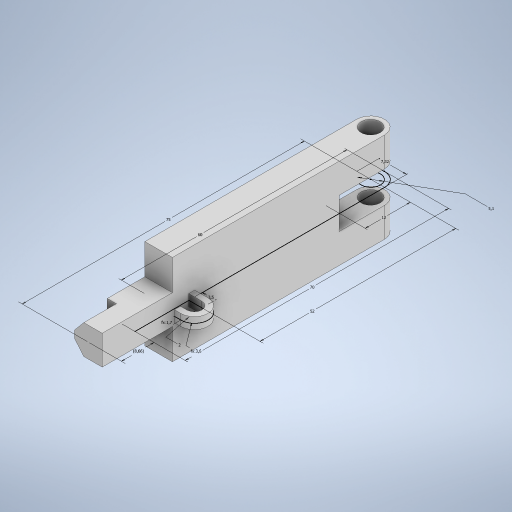
# Autodesk Inventor part: kredafullv3
Saved by Autodesk Inventor 2023 (Build 270158000, 158)
## iProperties
Created: 2023-03-10
Part Number: kredafullv3
Material: Ogólny
Document SubType Name: Modeling
Designer: kamil
Density: 1 g/cm^3
Appearance: Domyślna
Author: kamil
Autodesk Inventor part; units mm, degrees
ref_plane "YZ Plane" through (0, 0, 0) normal (1, 0, 0) x (0, 1, 0)
ref_plane "XZ Plane" through (0, 0, 0) normal (0, 1, 0) x (-1, 0, 0)
ref_plane "XY Plane" through (0, 0, 0) normal (0, 0, 1) x (1, 0, 0)
sketch "Szkic1" plane through (0, 0, 0) normal (0, 1, 0) x (-1, 0, 0)
  line L0 (-3.66, 66.34) -> (-3.66, 0)
  line L1 (-3.66, 0) -> (3.66, 0) construction
  line L2 (3.66, 0) -> (3.66, 66.34)
  arc A0 (-3.66, 0) -> (3.66, 0) centre (0, 0) ccw
  circle A1 centre (0, 0) radius 2.55
  line L3 (3.66, 12) -> (-3.66, 12)
  line L4 (3.66, 66.34) -> (-3.66, 66.34)
  line L5 (3.66, 56.34) -> (-3.66, 56.34)
  line L6 (0, 66.34) -> (0, 75) construction
  line L7 (-3.66, 52) -> (-7.16, 52)
  line L8 (-7.16, 52) -> (-7.16, 50.4)
  line L9 (-7.16, 50.4) -> (-3.66, 50.4)
  line L10 (-3.66, 50.4) -> (-3.66, 52)
  arc A2 (-7.16, 57.6) -> (-7.16, 50.4) centre (-7.16, 54) ccw
  arc A3 (-7.16, 56) -> (-7.16, 52) centre (-7.16, 54) ccw
  line L11 (-7.16, 57.6) -> (-5.46, 57.6)
  line L12 (-5.46, 57.6) -> (-5.46, 56)
  line L13 (-5.46, 56) -> (-7.16, 56)
  point P0 (0, -3.66)
  point P1 (0, 12)
  dimension "d0" = 7.32
  dimension "d3" = 5.1
  dimension "d17" = 12
  dimension "d26" = 70
  dimension "d27" = 60
  dimension "d30" = 75
  dimension "d31" = 8.66
  dimension "d35" = 2
  dimension "d36" = 3.6
  dimension "d37" = 3.5
  dimension "d38" = 1.7
  dimension "d39" = 52
  constraints: 28 end point, 7 point on circle, 6 tangent, 5 point on line, 4 centre point, 4 horizontal, 4 parallel, 3 coincident, 3 midpoint, 3 perpendicular, 1 concentric, 1 vertical, 1 vertical alignment
  measures "d0" distance between parallel lines of L0 L2
  measures "d3" diameter of A1
  measures "d17" distance of point (0, 0) point (0, 12)
  measures "d26" distance from line of point (0, -3.66) L4
  measures "d27" distance from line of point (0, -3.66) L5
  measures "d30" distance of point (0, 0) L6.end
  measures "d31" distance of L6.start L6.end
  measures "d35" radius of A3
  measures "d36" radius of A2
  measures "d37" distance of L8.end L9.end
  measures "d38" distance of L11.start L11.end
  measures "d39" distance of L7.start L0.end
extrude "Wyciągnięcie proste1" add sketch "Szkic1" along normal mid plane 24 contours L5 L2 L3 L0 | L2 A0 L0 L3
extrude "Wyciągnięcie proste4" cut sketch "Szkic1" along normal mid plane 8.35 contours L2 A0 L0 L3
extrude "Wyciągnięcie proste6" add sketch "Szkic1" along normal mid plane 7.8 contours L4 L2 L5 L0
sketch "Szkic4" plane through (-3.66, 3.9, 66.34) normal (0, 0, 1) x (1, 0, 0)
  line L0 (7.32, -7.8) -> (0, -7.8) projected
  line L1 (0, -7.8) -> (7.32, -7.8)
  line L2 (7.32, -7.8) -> (7.32, 0)
  line L3 (7.32, 0) -> (0, 0)
  line L4 (0, 0) -> (0, -7.8)
  line L5 (2.4334, -7.8) -> (0, -4.9)
  line L6 (0, 0.275) -> (0, -8.075) projected
  line L7 (0, -2.9) -> (2.4334, 0)
  line L8 (0, -3.9) -> (7.32, -3.9) construction
  point P0 (1.2167, -6.35)
  dimension "d43" = 50
  dimension "d44" = 2
  constraints: 14 end point, 4 point on line, 3 midpoint, 2 parallel, 1 horizontal, 1 perpendicular, 1 other
  measures "d43" angle of L0 L5
  measures "d44" distance of L5.end L7.start
extrude "Wyciągnięcie proste7" add sketch "Szkic4" along normal blind 8.66 contours L0 L5 L4 L7 L3 L2
extrude "Wyciągnięcie proste8" add sketch "Szkic1" along normal mid plane 3 contours L0 L9 L8 L7 | L8 A2 L11 L12 L13 A3
equation "\"d33\" = d31"
